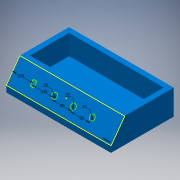
# Autodesk Inventor part: 240710_part2
Saved by Autodesk Inventor 2016 (Build 200138000, 138)
## iProperties
Created: 2024-07-10
Part Number: 240710_part2
Material: 일반
Document SubType Name: Modeling
Designer: pc
Density: 1 g/cm^3
Appearance: 기본값(1)
Author: pc
Autodesk Inventor part; units mm, degrees
ref_plane "YZ Plane" through (0, 0, 0) normal (1, 0, 0) x (0, 1, 0)
ref_plane "XZ Plane" through (0, 0, 0) normal (0, 1, 0) x (-1, 0, 0)
ref_plane "XY Plane" through (0, 0, 0) normal (0, 0, 1) x (1, 0, 0)
sketch "스케치1" plane through (0, 0, 0) normal (0, 0, 1) x (1, 0, 0)
  line L0 (250, -150) -> (-250, -150)
  line L1 (-250, -150) -> (-250, 150)
  line L2 (-250, 150) -> (250, 150)
  line L3 (250, 150) -> (250, -150)
  line L4 (250, -150) -> (-250, 150) construction
  line L5 (-250, -150) -> (250, 150) construction
  point P0 (0, 0)
  dimension "d0" = 500
  dimension "d1" = 300
  constraints: 12 end point, 2 midpoint, 2 parallel, 1 horizontal, 1 perpendicular
  measures "d0" distance of L1.end L2.end
  measures "d1" distance of L0.end L1.end
extrude "돌출1" add sketch "스케치1" along normal blind 120
sketch "스케치2" plane through (250, -150, 0) normal (1, 0, 0) x (0, 0, -1)
  line L0 (-120, 0) -> (-120, 300) projected
  line L1 (0, 0) -> (-120, 0) projected
  line L2 (-30, 0) -> (-120, 65)
  line L3 (-30, 0) -> (-30, -74.841)
  line L4 (-30, -74.841) -> (-182.9501, -91.3391)
  line L5 (-182.9501, -91.3391) -> (-221.4457, -10.4199)
  line L6 (-221.4457, -10.4199) -> (-120, 65)
  point P0 (0, 150)
  dimension "d4" = 65
  dimension "d5" = 30
  constraints: 10 end point, 2 point on line, 1 vertical
  measures "d4" distance of L2.end L0.start
  measures "d5" distance of L1.start L2.start
extrude "돌출2" cut sketch "스케치2" against normal through all contours L0 L2 L1
sketch "스케치3" plane through (0, 0, 120) normal (0, 0, 1) x (1, 0, 0)
  line L0 (-250, -85) -> (250, -85) projected
  line L1 (250, -85) -> (250, 150) projected
  line L2 (250, 150) -> (-250, 150) projected
  line L3 (-250, 150) -> (-250, -85) projected
  line L4 (-226, -61) -> (226, -61)
  line L5 (226, -61) -> (226, 126)
  line L6 (226, 126) -> (-226, 126)
  line L7 (-226, 126) -> (-226, -61)
  point P0 (0, 0)
  dimension "d8" = 24
  dimension "d9" = 24
  dimension "d10" = 24
  dimension "d11" = 24
  constraints: 8 end point, 2 parallel, 1 horizontal, 1 perpendicular
  measures "d8" distance between parallel lines of L3 L7
  measures "d9" distance between parallel lines of L2 L6
  measures "d10" distance between parallel lines of L0 L4
  measures "d11" distance between parallel lines of L1 L5
extrude "돌출3" cut sketch "스케치3" against normal blind 10 contours L7 L6 L5 L4
shell "쉘1" thickness 1.2 removed faces 5 at (75.3333, 1.3333, 110) at (-226, 63.6667, 116.6667) at (75.3333, 126, 116.6667) at (-75.3333, -61, 116.6667) at (226, 1.3333, 116.6667)
sketch "스케치4" plane through (0, 0, 120) normal (0, 0, 1) x (1, 0, 0)
  line L0 (-250, -85) -> (250, -85) projected
  line L1 (250, -85) -> (250, 150) projected
  line L2 (250, 150) -> (-250, 150) projected
  line L3 (-250, 150) -> (-250, -85) projected
  line L4 (-238, -73) -> (238, -73)
  line L5 (238, -73) -> (238, 138)
  line L6 (238, 138) -> (-238, 138)
  line L7 (-238, 138) -> (-238, -73)
  line L8 (-238, 32.5) -> (250, 32.5)
  line L9 (0, -73) -> (0, 138)
  point P0 (0, 0)
  dimension "d15" = 12
  dimension "d16" = 12
  dimension "d17" = 12
  dimension "d18" = 12
  constraints: 12 end point, 6 coincident, 4 midpoint, 2 parallel, 1 horizontal, 1 perpendicular
  measures "d15" distance between parallel lines of L0 L4
  measures "d16" distance between parallel lines of L3 L7
  measures "d17" distance between parallel lines of L2 L6
  measures "d18" distance between parallel lines of L1 L5
hole "구멍1" at (-238, -73, 120) at (-238, 138, 120) at (238, -73, 120) at (238, 138, 120) at (0, -73, 120) at (0, 138, 120) direction (0, 0, -1) diameter 4.134 depth 14.2 tip angle 118 thread size "M5x0.8" class "6H" standard "ISO Metric profile"
sketch "스케치5" plane through (-250, -150, 30) normal (0, -0.8106792, 0.5854906) x (1, 0, 0)
  line L0 (0, 0) -> (0, 111.018) projected
  line L1 (500, 0) -> (0, 0) projected
  line L2 (500, 111.018) -> (500, 0) projected
  line L3 (0, 111.018) -> (500, 111.018) projected
  circle A0 centre (200, 51.355) radius 12.5
  circle A1 centre (290, 51.355) radius 12.5
  circle A2 centre (380, 51.355) radius 12.5
  line L4 (109.038, 38.855) -> (90.962, 38.855)
  line L5 (90.962, 38.855) -> (90.962, 63.855)
  line L6 (90.962, 63.855) -> (109.038, 63.855)
  line L7 (109.038, 63.855) -> (109.038, 38.855)
  line L8 (109.038, 38.855) -> (90.962, 63.855) construction
  line L9 (90.962, 38.855) -> (109.038, 63.855) construction
  line L10 (455.4394, 12.1665) -> (493.5306, 12.1665) construction
  line L11 (493.5306, 12.1665) -> (493.5306, 2.974) construction
  line L12 (493.5306, 2.974) -> (455.4394, 2.974) construction
  line L13 (455.4394, 2.974) -> (455.4394, 12.1665) construction
  point P0 (250, 63.5032)
  point P1 (100, 51.355)
  dimension "d26" = 25
  dimension "d27" = 25
  dimension "d28" = 25
  dimension "d29" = 100
  dimension "d30" = 100
  dimension "d31" = 90
  dimension "d32" = 90
  constraints: 12 end point, 3 centre point, 2 midpoint, 2 parallel, 1 horizontal, 1 perpendicular, 2 other
  measures "d26" diameter of A0
  measures "d27" diameter of A1
  measures "d28" diameter of A2
  measures "d29" distance from line of L0 point (100, 51.355)
  measures "d30" distance of A0.centre point (100, 51.355)
  measures "d31" distance of A0.centre A1.centre
  measures "d32" distance of A2.centre A1.centre
sketch "스케치6" plane through (250, -150, 0) normal (1, 0, 0) x (0, 0, -1)
  line L0 (-120, 65) -> (-30, 0) projected
  line L1 (0, 0) -> (-30, 0) projected
  line L2 (0, 300) -> (0, 0) projected
  line L3 (0, 300) -> (-120, 300) projected
  line L4 (-120, 65) -> (-120, 300) projected
  point P0 (0, 150)
sketch "스케치7" plane through (250, -150, 0) normal (1, 0, 0) x (0, 0, -1)
  line L0 (-120, 65) -> (-30, 0) projected
  line L1 (0, 0) -> (-30, 0) projected
  line L2 (0, 300) -> (0, 0) projected
  line L3 (0, 300) -> (-120, 300) projected
  line L4 (-120, 65) -> (-120, 300) projected
  point P0 (0, 150)
